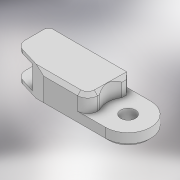
# Autodesk Inventor part: Upper Leg
Saved by Autodesk Inventor 2022 (Build 260153000, 153)
## iProperties
Created: 2022-02-25
Part Number: Upper Leg
Material: Generic
Document SubType Name: Modeling
Designer: joshw
Density: 1 g/cm^3
Appearance: Default
Author: joshw
Autodesk Inventor part; units mm, degrees
ref_plane "YZ Plane" through (0, 0, 0) normal (1, 0, 0) x (0, 1, 0)
ref_plane "XZ Plane" through (0, 0, 0) normal (0, 1, 0) x (-1, 0, 0)
ref_plane "XY Plane" through (0, 0, 0) normal (0, 0, 1) x (1, 0, 0)
sketch "Sketch2" plane through (0, 0, 0) normal (0, 1, 0) x (-1, 0, 0)
  line L0 (-5.5536, -11.7431) -> (5.5568, -15.0764)
  line L1 (5.5568, -25.2431) -> (-23.9154, -25.2431)
  line L2 (-23.9154, -25.2431) -> (-23.9154, -11.7431)
  line L3 (-5.5536, -11.7431) -> (-23.9154, -11.7431)
  line L4 (5.5568, -25.2431) -> (5.5568, -15.0764)
  circle A0 centre (-23.9154, -18.4931) radius 6.75
  circle A1 centre (-23.9154, -18.4931) radius 2.2
  circle A2 centre (-23.9154, -18.4931) radius 6.202
  circle A3 centre (-24.9154, -18.9931) radius 6.25
  line L5 (-18.8553, -31.0955) -> (-18.419, -3.4058)
  point P0 (0, 0)
  point P1 (0, 0)
  point P2 (-19.4912, -10.8803)
  point P3 (-19.4912, -24.3803)
  point P4 (-23.9154, -12.2912)
  point P5 (-23.9154, -24.6951)
  dimension "d1" = 13.5
  dimension "d0" = 4.4
  dimension "d6" = 0.5
  dimension "d7" = 1
  dimension "d8" = 12.5
  constraints: 12 end point, 3 centre point, 3 coincident, 2 horizontal, 2 vertical, 1 midpoint, 1 tangent, 3 other
  measures "d0" diameter of A1
  measures "d6" vertical distance of point (-23.915, -18.493) point (-24.915, -18.993)
  measures "d7" horizontal distance of point (-23.915, -18.493) point (-24.915, -18.993)
  measures "d8" diameter of A3
extrude "Extrusion1" add sketch "Sketch2" along normal blind 3.85 contours L0 L4 L1 L5 A0 L3 | L5 A0 L3 | A0 L5 A2 L2 | L2 A2 A3 A0 | A0 L5 A2 | L1 A0 L5 | A2 L5 A3 L2 | L2 A3 A2 | A3 A2 L2 A0 | L5 A2 A3 | A2 L5 | A0 A3 L2 | L2 A3 A2 L5 A0 | A3 A2 L2 A1 | L2 A1 A2 A3 | L2 A2 A3
extrude "Extrusion2" add sketch "Sketch2" along normal blind 8.85 contours L0 L4 L1 L5 A0 L3 | L5 A0 L3 | A0 L5 A2 L2 | A0 L5 A2 | L1 A0 L5 | L2 A3 A2 L5 A0 | L2 A2 A3 picked at (-23.6214, -24.9369)
sketch "Sketch3" plane through (0, 8.85, 0) normal (0, 1, 0) x (1, 0, 0)
  line L0 (-5.5568, 25.2431) -> (-5.5568, 15.0764) projected
  line L1 (-5.5568, 15.0764) -> (5.5536, 11.7431) projected
  line L2 (5.5536, 11.7431) -> (23.9154, 11.7431) projected
  line L3 (23.9154, 11.7431) -> (23.9154, 12.2912) projected
  arc A0 (23.9154, 24.6951) -> (23.9154, 12.2912) centre (23.9154, 18.4931) ccw projected
  line L4 (23.9154, 24.6951) -> (23.9154, 25.2431) projected
  line L5 (23.9154, 25.2431) -> (-5.5568, 25.2431) projected
  line L6 (18.8553, 31.0955) -> (18.419, 3.4058) projected
  point P0 (0, 0)
  point P1 (18.6062, 15.2873)
  point P2 (18.5504, 11.7431)
  point P3 (18.7631, 25.2431)
  point P4 (18.7099, 21.8646)
extrude "Extrusion3" cut sketch "Sketch3" against normal up to surface (5 mm away) contours L5 L4 A0 L6 | L6 A0 L3 L2
sketch "Sketch4" plane through (-5.5568, 0, -25.2431) normal (-1, 0, 0) x (0, 0, 1)
  line L0 (0, 0) -> (10.1667, 0) projected
  line L1 (10.1667, 0) -> (10.1667, 8.85) projected
  line L2 (0, 8.85) -> (10.1667, 8.85) projected
  line L3 (0, 0) -> (0, 8.85) projected
  line L4 (9.1667, 7.85) -> (9.1667, 1)
  line L5 (9.1667, 1) -> (1, 1)
  line L6 (1, 1) -> (1, 7.85)
  line L7 (1, 7.85) -> (9.1667, 7.85)
  point P0 (25.2431, 0)
  dimension "d11" = 1
  constraints: 8 end point, 3 other
  measures "d11" distance between parallel lines of L2 L7
extrude "Extrusion4" cut sketch "Sketch4" against normal blind 8 contours L4 L5 L6 L7
sketch "Sketch5" plane through (-5.5568, 1, -16.0764) normal (0, 1, 0) x (1, 0, 0)
  line L0 (0, 0) -> (0, 8.1667) projected
  line L1 (0, 0) -> (8, 0) projected
  line L2 (8, 0) -> (8, 8.1667) projected
  line L3 (0, 8.1667) -> (8, 8.1667) projected
  line L4 (8, 4.0834) -> (2.9855, 4.0834) construction
  line L5 (4, 0) -> (4, 4.0834) construction
  circle A0 centre (4, 4.0834) radius 2.55
  point P0 (5.5568, -16.0764)
  dimension "d14" = 5.1
  constraints: 4 end point, 2 midpoint, 1 centre point, 1 coincident, 1 horizontal, 1 perpendicular, 1 point on line
  measures "d14" diameter of A0
extrude "Extrusion5" add sketch "Sketch5" along normal up to surface (6.85 mm away) contours A0
sketch "Sketch6" plane through (5.5536, 0, -11.7431) normal (0, 0, 1) x (1, 0, 0)
  line L0 (-11.1104, 7.85) -> (-11.1104, 1) projected
  line L1 (-11.1104, 7.85) -> (-4.8007, 7.85)
  line L2 (-4.8007, 7.85) -> (-4.8007, 1)
  line L3 (-11.1104, 1) -> (-4.8007, 1)
  point P0 (-5.5536, 0)
  constraints: 6 end point
extrude "Extrusion6" cut sketch "Sketch6" against normal up to surface (4.3333 mm away)
sketch "Sketch7" plane through (-5.5568, 1, -24.2431) normal (0, 0, 1) x (1, 0, 0)
  line L0 (0, 0) -> (0, 6.85) projected
  line L1 (0, 0) -> (8, 0) projected
  line L2 (8, 0) -> (8, 6.85) projected
  line L3 (0, 6.85) -> (8, 6.85) projected
  point P0 (5.5568, -1)
extrude "Extrusion7" cut sketch "Sketch7" against normal blind 10.25
sketch "Sketch8" plane through (0, 8.85, 0) normal (0, 1, 0) x (1, 0, 0)
  circle A0 centre (-1.5568, 20.1598) radius 2.55 projected
  circle A1 centre (-1.5568, 20.1598) radius 2.55 projected
  line L0 (-5.5568, 25.2431) -> (2.4432, 25.2431) projected
  point P0 (0, 0)
fillet "Fillet1" radius 3 2 edges at (-5.5568, 8.35, -15.0764) (-5.5568, 0.5, -15.0764)
chamfer "Chamfer1" distance 2 angle 45 2 edges at (-5.5568, 8.35, -25.2431) (-5.5568, 0.5, -25.2431)
chamfer "Chamfer2" distance 2 angle 45 1 edges at (18.7631, 6.35, -25.2431)
fillet "Fillet2" radius 3 1 edges at (18.5504, 6.35, -11.7431)
chamfer "Chamfer3" distance 1 angle 45 7 edges at (6.6031, 8.85, -25.2431) (10.5754, 8.85, -11.7431) (17.7018, 8.85, -12.6052) (18.6016, 8.85, -14.9916) (14.7345, 0, -11.7431) (30.6654, 0, -18.4931) (10.1793, 0, -25.2431)
body "Solid1"
